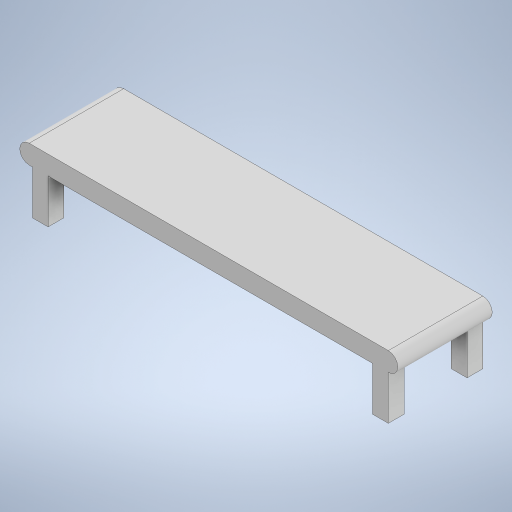
# Autodesk Inventor part: SoporteBanda
Saved by Autodesk Inventor 2024 (Build 280153000, 153)
## iProperties
Created: 2024-06-27
Part Number: SoporteBanda
Material: Genérico
Document SubType Name: Modeling
Designer: USER
Density: 1 g/cm^3
Appearance: Valor por defecto
Author: USER
Autodesk Inventor part; units mm, degrees
ref_plane "YZ Plane" through (0, 0, 0) normal (1, 0, 0) x (0, 1, 0)
ref_plane "XZ Plane" through (0, 0, 0) normal (0, 1, 0) x (-1, 0, 0)
ref_plane "XY Plane" through (0, 0, 0) normal (0, 0, 1) x (1, 0, 0)
sketch "Boceto1" plane through (0, 0, 0) normal (0, 1, 0) x (-1, 0, 0)
  line L0 (3000, -750) -> (-3000, -750)
  line L1 (-3000, -750) -> (-3000, 750)
  line L2 (-3000, 750) -> (3000, 750)
  line L3 (3000, 750) -> (3000, -750)
  line L4 (3000, -750) -> (-3000, 750) construction
  line L5 (-3000, -750) -> (3000, 750) construction
  point P0 (0, 0)
  dimension "d0" = 6000
  dimension "d1" = 1500
  constraints: 12 end point, 2 midpoint, 2 parallel, 1 horizontal, 1 perpendicular
  measures "d0" distance of L1.end L2.end
  measures "d1" distance between parallel lines of L0 L2
extrude "Extrusión1" add sketch "Boceto1" along normal blind 300
sketch "Boceto2" plane through (-3000, 0, 750) normal (0, 0, 1) x (1, 0, 0)
  line L0 (6000, 0) -> (6000, 300) projected
  line L1 (0, 300) -> (6000, 300) projected
  line L2 (0, 0) -> (6000, 0) projected
  line L3 (0, 0) -> (0, 300) projected
  circle A0 centre (5850, 150) radius 150
  circle A1 centre (150, 150) radius 150
  line L4 (5850, 300) -> (6000, 300)
  line L5 (6000, 0) -> (5850, 0)
  line L6 (150, 0) -> (0, 0)
  line L7 (0, 300) -> (150, 300)
  line L8 (0, 0) -> (0, 300)
  line L9 (6000, 0) -> (6000, 300)
  point P0 (3000, 0)
  point P1 (6000, 150)
  point P2 (0, 150)
  constraints: 12 end point, 8 tangent, 4 point on circle, 4 point on line, 3 collinear, 2 centre point, 1 parallel
extrude "Extrusión2" cut sketch "Boceto2" against normal through all contours L2 A0 L0 | A0 L1 L0 | L2 L3 A1 | A1 L3 L1
sketch "Boceto3" plane through (0, 0, 0) normal (0, -1, 0) x (1, 0, 0)
  line L0 (-2850, 750) -> (2850, 750) projected
  line L1 (2850, -750) -> (2850, 750) projected
  line L2 (2850, -750) -> (-2850, -750) projected
  line L3 (-2850, -750) -> (-2850, 750) projected
  line L4 (2850, 750) -> (2850, 500)
  line L5 (2850, 500) -> (2600, 500)
  line L6 (2600, 500) -> (2600, 750)
  line L7 (2600, 750) -> (2850, 750)
  line L8 (2850, -500) -> (2850, -750)
  line L9 (2850, -750) -> (2600, -750)
  line L10 (2600, -750) -> (2600, -500)
  line L11 (2600, -500) -> (2850, -500)
  line L12 (-2550, 750) -> (-2550, 500)
  line L13 (-2550, 500) -> (-2800, 500)
  line L14 (-2800, 500) -> (-2800, 750)
  line L15 (-2800, 750) -> (-2550, 750)
  line L16 (-2550, -500) -> (-2550, -750)
  line L17 (-2550, -750) -> (-2800, -750)
  line L18 (-2800, -750) -> (-2800, -500)
  line L19 (-2800, -500) -> (-2550, -500)
  point P0 (0, 0)
  point P1 (2600, 750)
  point P2 (2600, -750)
  point P3 (-2800, 750)
  point P4 (-2800, -750)
  point P5 (-2550, -750)
  dimension "d6" = 250
  dimension "d7" = 250
  dimension "d10" = 1250
  dimension "d13" = 5400
  constraints: 32 end point, 2 parallel, 1 horizontal, 1 perpendicular, 1 point on line, 1 vertical, 24 other
  measures "d6" distance of L0.end L4.end
  measures "d7" distance of L4.end L5.end
  measures "d10" distance of L4.end L8.end
  measures "d13" distance of L4.end L12.end
extrude "Extrusión3" add sketch "Boceto3" along normal blind 700 contours L0 L12 L13 L14 | L18 L19 L16 L2 | L0 L1 L5 L6 | L10 L11 L1 L2
equation "\"d0\" = L"
equation "\"L\" = 6000"
